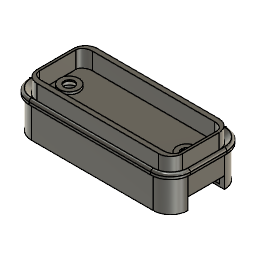
Modul na widgety (Autodesk Fusion 360 design; units mm, degrees)
Autodesk Fusion 360 part; units mm, degrees
note: some values were not read from the file. Set by a fixed rule: which sketch regions a step uses.
sketch "Sketch1" plane through (0, 0, 0) normal (0, 0, 1) x (1, 0, 0)
  line L0 (25, 12.5) -> (-25, 12.5)
  line L1 (-30, 7.5) -> (-30, -7.5)
  line L2 (-25, -12.5) -> (25, -12.5)
  line L3 (30, -7.5) -> (30, 7.5)
  line L4 (-30, 12.5) -> (30, -12.5) construction
  line L5 (-30, -12.5) -> (30, 12.5) construction
  arc A0 (-25, 12.5) -> (-30, 7.5) centre (-25, 7.5) ccw
  arc A1 (30, 7.5) -> (25, 12.5) centre (25, 7.5) ccw
  arc A2 (25, -12.5) -> (30, -7.5) centre (25, -7.5) ccw
  arc A3 (-30, -7.5) -> (-25, -12.5) centre (-25, -7.5) ccw
  circle A4 centre (-24.15, 0) radius 4.85
  line L6 (-30, 0) -> (30, 0) construction
  line L7 (-30, 0) -> (-29, 0) construction
  line L8 (0, 1.75) -> (0, 22.5) construction
  circle A5 centre (24.15, 0) radius 4.85
  circle A6 centre (-24.15, 0) radius 1.75
  circle A7 centre (24.15, 0) radius 1.75
  line L9 (29, -7.5) -> (29, 7.5)
  arc A8 (29, 7.5) -> (25, 11.5) centre (25, 7.5) ccw
  line L10 (25, 11.5) -> (-25, 11.5)
  arc A9 (-25, 11.5) -> (-29, 7.5) centre (-25, 7.5) ccw
  line L11 (-29, 7.5) -> (-29, -7.5)
  arc A10 (-29, -7.5) -> (-25, -11.5) centre (-25, -7.5) ccw
  line L12 (-25, -11.5) -> (25, -11.5)
  arc A11 (25, -11.5) -> (29, -7.5) centre (25, -7.5) ccw
  dimension "d10" = 60
  dimension "d11" = 25
  dimension "d12" = 5
  dimension "d15" = 9.7
  dimension "d16" = 1
  dimension "d17" = 3.5
  dimension "d20" = -1
  constraint horizontal L0
  constraint vertical L1
  constraint horizontal L2
  constraint vertical L3
  constraint midpoint L5 origin
  constraint coincident L4.start L1
  constraint coincident L4.start L0
  constraint tangent L1 A0
  constraint tangent L0 A0
  constraint coincident L5.end L0
  constraint coincident L5.end L3
  constraint tangent L0 A1
  constraint tangent L3 A1
  constraint equal A0 A1
  constraint coincident L4.end L3
  constraint coincident L4.end L2
  constraint tangent L3 A2
  constraint tangent L2 A2
  constraint equal A0 A2
  constraint coincident L5.start L2
  constraint coincident L5.start L1
  constraint tangent L2 A3
  constraint tangent L1 A3
  constraint equal A0 A3
  constraint midpoint L1 L6.start
  constraint midpoint L3 L6.end
  constraint coincident A4.centre L6
  constraint coincident A4 L7.end
  constraint coincident L6 L7.end
  constraint symmetric A4 L8 A5
  constraint concentric A4 A6
  constraint symmetric L8 A6 A7
  measures "d10" distance of L5.end L4.start
  measures "d11" distance of L4.start L5.start
  measures "d12" radius of A0
  measures "d15" diameter of A4
  measures "d16" distance of L6.start L7.end
  measures "d17" diameter of A6
extrude "Extrude1" add sketch "Sketch1" along normal blind 4.6 contours L0 L1 L2 L3 A0 A1 A2 A3 | L9 A8 L10 A9 L11 A10 L12 A11 makes body 1
extrude "Extrude2" add sketch "Sketch1" along normal blind 1 contours A4 | A5 bodies 1
extrude "Extrude3" add sketch "Sketch1" against normal blind 3.9 contours L0 L1 L2 L3 A0 A1 A2 A3 bodies 1
extrude "Extrude4" cut 1 faces at (29, -2.5, -1.3) along direction (1, 0, 0) blind 2 on bodies 1 bodies 1
extrude "Extrude5" cut 1 faces at (-29, 2.5, -1.3) along direction (-1, 0, 0) blind 3 on bodies 1 bodies 1
move_face "OffsetFaces1" offset 4 6 faces at (-27.4726, -10.6442, -2.6) (-8.3333, -11.5, -1.3) (28.2583, -9.8202, -2.6) (27.7603, 10.3949, -2.6) (8.3333, 11.5, -1.3) (-27.7603, 10.3949, -2.6) on bodies 1
copy_body "Body->Comp1" bodies 1 removing the originals makes body 2 in component "spodní část nasazovací"
sketch "Sketch1 (2)" plane through (0, 0, -3.9) normal (0, 0, -1) x (1, 0, 0) in component "spodní část hlavní"
  line L0 (30, -7.5) -> (-30, -7.5)
  arc A0 (-30, -7.5) -> (-25, -12.5) centre (-25, -7.5) ccw
  line L1 (-25, -12.5) -> (25, -12.5)
  arc A1 (25, -12.5) -> (30, -7.5) centre (25, -7.5) ccw
  line L2 (-30, -7.5) -> (30, -7.5)
  line L3 (30, -7.5) -> (30, 7.5)
  line L4 (30, 7.5) -> (-30, 7.5)
  line L5 (-30, 7.5) -> (-30, -7.5)
  circle A2 centre (24.15, 0) radius 1.75
  circle A3 centre (-24.15, 0) radius 1.75
  line L6 (-30, 7.5) -> (30, 7.5)
  arc A4 (30, 7.5) -> (25, 12.5) centre (25, 7.5) ccw
  line L7 (25, 12.5) -> (-25, 12.5)
  arc A5 (-25, 12.5) -> (-30, 7.5) centre (-25, 7.5) ccw
extrude "Extrude1'" add sketch "Sketch1 (2)" along normal blind 1 separate body contours L0 A0 L1 A1 L2 | L0 L2 L3 L4 L5 L6 | L4 L6 A4 L7 A5 | A2 | A3 makes body 3 in component "spodní část hlavní"
sketch "Sketch2" plane through (0, 0, -4.9) normal (0, 0, -1) x (1, 0, 0) in component "spodní část hlavní"
  arc A0 (-25, 12.5) -> (-30, 7.5) centre (-25, 7.5) ccw
  line L0 (-30, 7.5) -> (-30, -7.5)
  arc A1 (-30, -7.5) -> (-25, -12.5) centre (-25, -7.5) ccw
  line L1 (-25, -12.5) -> (25, -12.5)
  arc A2 (25, -12.5) -> (30, -7.5) centre (25, -7.5) ccw
  line L2 (30, -7.5) -> (30, 7.5)
  arc A3 (30, 7.5) -> (25, 12.5) centre (25, 7.5) ccw
  line L3 (25, 12.5) -> (-25, 12.5)
  line L4 (-30.15, 7.5) -> (-30.15, -7.5)
  arc A4 (-30.15, -7.5) -> (-25, -12.65) centre (-25, -7.5) ccw
  line L5 (-25, -12.65) -> (25, -12.65)
  arc A5 (25, -12.65) -> (30.15, -7.5) centre (25, -7.5) ccw
  line L6 (30.15, -7.5) -> (30.15, 7.5)
  arc A6 (30.15, 7.5) -> (25, 12.65) centre (25, 7.5) ccw
  line L7 (25, 12.65) -> (-25, 12.65)
  arc A7 (-25, 12.65) -> (-30.15, 7.5) centre (-25, 7.5) ccw
  line L8 (-32.15, 7.5) -> (-32.15, -7.5)
  arc A8 (-32.15, -7.5) -> (-25, -14.65) centre (-25, -7.5) ccw
  line L9 (-25, -14.65) -> (25, -14.65)
  arc A9 (25, -14.65) -> (32.15, -7.5) centre (25, -7.5) ccw
  line L10 (32.15, -7.5) -> (32.15, 7.5)
  arc A10 (32.15, 7.5) -> (25, 14.65) centre (25, 7.5) ccw
  line L11 (25, 14.65) -> (-25, 14.65)
  arc A11 (-25, 14.65) -> (-32.15, 7.5) centre (-25, 7.5) ccw
  line L12 (30, 7.5) -> (32.15, 7.5)
  line L13 (30, -7.5) -> (32.15, -7.5)
  line L14 (-30, -7.5) -> (-32.15, -7.5)
  line L15 (-30, 7.5) -> (-32.15, 7.5)
  dimension "d30" = 0.15
  dimension "d31" = 2
  constraint coincident L2.end A3.start
  constraint perpendicular L10 L12
  constraint coincident A2.end L2.start
  constraint perpendicular L10 L13
  constraint coincident L0.end A1.start
  constraint perpendicular L8 L14
  constraint coincident A0.end L0.start
  constraint perpendicular L8 L15
extrude "Extrude2'" add sketch "Sketch2" against normal blind 1 contours A0 A3 L3 A6 L7 A7 L12 L15 | L0 L4 L14 L15 | A1 L1 A2 A4 L5 A5 L13 L14 | A6 L7 A7 A10 L11 A11 L12 L15 | L4 L8 L14 L15 | L2 L6 L12 L13 | A4 L5 A5 A8 L9 A9 L13 L14 | L6 L10 L12 L13 bodies 3 in component "spodní část hlavní"
extrude "Extrude3'" add sketch "Sketch2" against normal blind 13.2 contours A6 L7 A7 A10 L11 A11 L12 L15 | L4 L8 L14 L15 | A4 L5 A5 A8 L9 A9 L13 L14 | L6 L10 L12 L13 bodies 3 in component "spodní část hlavní"
sketch "Sketch3" plane through (0, 0, 8.3) normal (0, 0, 1) x (-1, 0, 0) in component "spodní část hlavní"
  arc A0 (30.15, 7.5) -> (25, 12.65) centre (25, 7.5) ccw
  line L0 (30.15, 7.5) -> (30.15, -7.5)
  arc A1 (25, -12.65) -> (30.15, -7.5) centre (25, -7.5) ccw
  line L1 (25, -12.65) -> (-25, -12.65)
  arc A2 (-30.15, -7.5) -> (-25, -12.65) centre (-25, -7.5) ccw
  line L2 (-30.15, -7.5) -> (-30.15, 7.5)
  arc A3 (-25, 12.65) -> (-30.15, 7.5) centre (-25, 7.5) ccw
  line L3 (-25, 12.65) -> (25, 12.65)
  arc A4 (32.15, 7.5) -> (25, 14.65) centre (25, 7.5) ccw
  line L4 (25, 14.65) -> (-25, 14.65)
  arc A5 (-25, 14.65) -> (-32.15, 7.5) centre (-25, 7.5) ccw
  line L5 (-32.15, 7.5) -> (-32.15, -7.5)
  arc A6 (-32.15, -7.5) -> (-25, -14.65) centre (-25, -7.5) ccw
  line L6 (-25, -14.65) -> (25, -14.65)
  arc A7 (25, -14.65) -> (32.15, -7.5) centre (25, -7.5) ccw
  line L7 (32.15, -7.5) -> (32.15, 7.5)
  arc A8 (-33.15, -7.5) -> (-25, -15.65) centre (-25, -7.5) ccw
  line L8 (-25, -15.65) -> (25, -15.65)
  arc A9 (25, -15.65) -> (33.15, -7.5) centre (25, -7.5) ccw
  line L9 (33.15, -7.5) -> (33.15, 7.5)
  arc A10 (33.15, 7.5) -> (25, 15.65) centre (25, 7.5) ccw
  line L10 (25, 15.65) -> (-25, 15.65)
  arc A11 (-25, 15.65) -> (-33.15, 7.5) centre (-25, 7.5) ccw
  line L11 (-33.15, 7.5) -> (-33.15, -7.5)
  dimension "d36" = 1
extrude "Extrude4'" add sketch "Sketch3" along normal blind 2 contours A4 L4 A5 L5 A6 L6 A7 L7 | A8 L8 A9 L9 A10 L10 A11 L11 bodies 3 in component "spodní část hlavní"
chamfer "Chamfer1" distance 2 angle 45 8 edges at (30.15, 0, 10.3) (28.6416, -11.1416, 10.3) (0, -12.65, 10.3) (-28.6416, -11.1416, 10.3) (-30.15, 0, 10.3) (-28.6416, 11.1416, 10.3) (0, 12.65, 10.3) (28.6416, 11.1416, 10.3) on bodies 3 in component "spodní část hlavní"
fillet "Fillet1" radius 1 8 edges at (0, 15.65, 10.3) (-30.7629, 13.2629, 10.3) (-33.15, 0, 10.3) (-30.7629, -13.2629, 10.3) (0, -15.65, 10.3) (30.7629, -13.2629, 10.3) (33.15, 0, 10.3) (30.7629, 13.2629, 10.3) on bodies 3 in component "spodní část hlavní"
extrude "Extrude5'" cut sketch "Sketch1" against normal blind 14 contours A4 | A5 | L9 A8 L10 A9 L11 A10 L12 A11 | A6 | A7 bodies 3 in component "spodní část hlavní"
extrude "Extrude6" add 2 faces at (8.3333, -9.1667, -3.9) (8.3333, 9.1667, -3.9) along direction (0, 0, -1) blind 1 on bodies 2 bodies 3 in component "spodní část hlavní"
sketch "Sketch4" plane through (0, 0, -4.9) normal (0, 0, -1) x (1, 0, 0) in component "spodní část hlavní"
  line L0 (-29, -7.5) -> (-29, 7.5)
  line L1 (-29, 7.5) -> (29, 7.5)
  line L2 (29, 7.5) -> (29, -7.5)
  line L3 (29, -7.5) -> (-29, -7.5)
  arc A0 (-25, 14.65) -> (-32.15, 7.5) centre (-25, 7.5) ccw
  line L4 (-32.15, 7.5) -> (-32.15, -7.5)
  arc A1 (-32.15, -7.5) -> (-25, -14.65) centre (-25, -7.5) ccw
  line L5 (-25, -14.65) -> (25, -14.65)
  arc A2 (25, -14.65) -> (32.15, -7.5) centre (25, -7.5) ccw
  line L6 (32.15, -7.5) -> (32.15, 7.5)
  arc A3 (32.15, 7.5) -> (25, 14.65) centre (25, 7.5) ccw
  line L7 (25, 14.65) -> (-25, 14.65)
  line L8 (-29, -7.5) -> (-32.15, -7.5)
  line L9 (-29, 7.5) -> (-32.15, 7.5)
  line L10 (29, -7.5) -> (32.15, -7.5)
  line L11 (29, 7.5) -> (32.15, 7.5)
  constraint coincident L0.start L3.end
  constraint coincident L4.end A1.start
  constraint coincident L0.end L1.start
  constraint coincident A0.end L4.start
  constraint coincident L2.end L3.start
  constraint coincident A2.end L6.start
  constraint coincident L1.end L2.start
  constraint coincident L6.end A3.start
extrude "Extrude7" cut sketch "Sketch4" against normal blind 4.9 contours L0 L4 L8 L9 | L2 L6 L10 L11 bodies 3 in component "spodní část hlavní"
sketch "Sketch1 (3)" plane through (0, 0, 4.6) normal (0, 0, 1) x (-1, 0, 0) in component "stejná část widgetu"
  circle A0 centre (24.15, 0) radius 4.85
  circle A1 centre (-24.15, 0) radius 4.85
  arc A2 (-30, -7.5) -> (-25, -12.5) centre (-25, -7.5) ccw
  line L0 (-25, -12.5) -> (25, -12.5)
  arc A3 (25, -12.5) -> (30, -7.5) centre (25, -7.5) ccw
  line L1 (30, -7.5) -> (30, 7.5)
  arc A4 (30, 7.5) -> (25, 12.5) centre (25, 7.5) ccw
  line L2 (25, 12.5) -> (-25, 12.5)
  arc A5 (-25, 12.5) -> (-30, 7.5) centre (-25, 7.5) ccw
  line L3 (-30, 7.5) -> (-30, -7.5)
  circle A6 centre (-24.15, 0) radius 3.8
  circle A7 centre (-24.15, 0) radius 2.15
  line L4 (0, -2.5) -> (0, -20)
  circle A8 centre (24.15, 0) radius 2.15
  circle A9 centre (24.15, 0) radius 3.8
  line L5 (-25, -12.45) -> (25, -12.45)
  arc A10 (25, -12.45) -> (29.95, -7.5) centre (25, -7.5) ccw
  line L6 (29.95, -7.5) -> (29.95, 7.5)
  arc A11 (29.95, 7.5) -> (25, 12.45) centre (25, 7.5) ccw
  line L7 (25, 12.45) -> (-25, 12.45)
  arc A12 (-25, 12.45) -> (-29.95, 7.5) centre (-25, 7.5) ccw
  line L8 (-29.95, 7.5) -> (-29.95, -7.5)
  arc A13 (-29.95, -7.5) -> (-25, -12.45) centre (-25, -7.5) ccw
  dimension "d48" = 7.6
  dimension "d49" = 4.3
  dimension "d65" = -0.05
  constraint concentric A1 A6
  constraint concentric A6 A7
  constraint symmetric A6 L4 A9
  constraint symmetric A7 L4 A8
  measures "d48" diameter of A6
  measures "d49" diameter of A7
extrude "Extrude1''" add sketch "Sketch1 (3)" along normal blind 3.2 separate body contours A0 | A1 | A6 | A9 | L5 A10 L6 A11 L7 A12 L8 A13 makes body 4 in component "stejná část widgetu"
chamfer "Chamfer1'" distance 3.2 distance2 1.65 2 edges at (26.1545, -0.7775, 4.6) (-22.1455, -0.7775, 4.6) measured on face at (22.0027, 0.1072, 6.7333) measured on face at (-26.2973, 0.1072, 6.7333) on bodies 4 in component "stejná část widgetu"
sketch "Sketch2 (2)" plane through (0, 0, 4.6) normal (0, 0, -1) x (1, 0, 0) in component "stejná část widgetu"
  circle A0 centre (24.15, 0) radius 3.8
  circle A1 centre (-24.15, 0) radius 3.8
  arc A2 (25, -12.45) -> (29.95, -7.5) centre (25, -7.5) ccw
  line L0 (29.95, -7.5) -> (29.95, 7.5)
  arc A3 (29.95, 7.5) -> (25, 12.45) centre (25, 7.5) ccw
  line L1 (25, 12.45) -> (-25, 12.45)
  arc A4 (-25, 12.45) -> (-29.95, 7.5) centre (-25, 7.5) ccw
  line L2 (-29.95, 7.5) -> (-29.95, -7.5)
  arc A5 (-29.95, -7.5) -> (-25, -12.45) centre (-25, -7.5) ccw
  line L3 (-25, -12.45) -> (25, -12.45)
extrude "Extrude2''" cut sketch "Sketch2 (2)" against normal blind 1 contours A0 | A1 | A2 L0 A3 L1 A4 L2 A5 L3 bodies 4 in component "stejná část widgetu"
extrude "Extrude3''" add 1 faces at (-7.4043, -8.611, 7.8) along direction (0, 0, 1) blind 0.5 on bodies 4 bodies 4 in component "stejná část widgetu"
sketch "Sketch3 (2)" plane through (0, 0, 8.3) normal (0, 0, 1) x (-1, 0, 0) in component "stejná část widgetu"
  circle A0 centre (24.15, 0) radius 2.15
  circle A1 centre (-24.15, 0) radius 2.15
  circle A2 centre (-24.15, 0) radius 4
  line L0 (0, -2.5) -> (0, -20)
  circle A3 centre (24.15, 0) radius 4
  arc A4 (-29.95, -7.5) -> (-25, -12.45) centre (-25, -7.5) ccw
  line L1 (-25, -12.45) -> (25, -12.45)
  arc A5 (25, -12.45) -> (29.95, -7.5) centre (25, -7.5) ccw
  line L2 (29.95, -7.5) -> (29.95, 7.5)
  arc A6 (29.95, 7.5) -> (25, 12.45) centre (25, 7.5) ccw
  line L3 (25, 12.45) -> (-25, 12.45)
  arc A7 (-25, 12.45) -> (-29.95, 7.5) centre (-25, 7.5) ccw
  line L4 (-29.95, 7.5) -> (-29.95, -7.5)
  dimension "d58" = 8
  constraint concentric A1 A2
  constraint symmetric A2 L0 A3
  measures "d58" diameter of A2
extrude "Extrude4''" cut sketch "Sketch3 (2)" against normal blind 1 contours A4 L1 A5 L2 A6 L3 A7 L4 bodies 4 in component "stejná část widgetu"
sketch "Sketch4 (2)" plane through (0, 0, 7.3) normal (0, 0, 1) x (-1, 0, 0) in component "stejná část widgetu"
  circle A0 centre (24.15, 0) radius 4
  circle A1 centre (-24.15, 0) radius 4
  line L0 (-29.95, 7.5) -> (-29.95, -7.5)
  arc A2 (-29.95, -7.5) -> (-25, -12.45) centre (-25, -7.5) ccw
  line L1 (-25, -12.45) -> (25, -12.45)
  arc A3 (25, -12.45) -> (29.95, -7.5) centre (25, -7.5) ccw
  line L2 (29.95, -7.5) -> (29.95, 7.5)
  arc A4 (29.95, 7.5) -> (25, 12.45) centre (25, 7.5) ccw
  line L3 (25, 12.45) -> (-25, 12.45)
  arc A5 (-25, 12.45) -> (-29.95, 7.5) centre (-25, 7.5) ccw
  line L4 (-25, -10.45) -> (25, -10.45)
  line L5 (25, 10.45) -> (-25, 10.45)
  line L6 (-28.95, 7.5) -> (-28.95, -7.5)
  line L7 (28.95, -7.5) -> (28.95, 7.5)
  spline S0 degree 5 poles (-25, 10.45) (-25.2273, 10.45) (-25.6786, 10.4247) (-26.3452, 10.3108) (-27.2024, 10.0207) (-28.141, 9.4513) (-28.6824, 8.8161) (-28.9013, 8.2133) (-28.95, 7.7483) (-28.95, 7.5) knots 0 0 0 0 0 0 0.2 0.4 0.6 0.8 1 1 1 1 1 1
  spline S1 degree 5 poles (-28.95, -7.5) (-28.95, -7.7625) (-28.9031, -8.2507) (-28.6924, -8.8725) (-28.1699, -9.5067) (-27.2532, -10.0523) (-26.3968, -10.3218) (-25.7128, -10.4267) (-25.2404, -10.45) (-25, -10.45) knots 0 0 0 0 0 0 0.2 0.4 0.6 0.8 1 1 1 1 1 1
  spline S2 degree 5 poles (25, -10.45) (25.2273, -10.45) (25.6786, -10.4247) (26.3452, -10.3108) (27.2024, -10.0207) (28.141, -9.4513) (28.6824, -8.8161) (28.9013, -8.2133) (28.95, -7.7483) (28.95, -7.5) knots 0 0 0 0 0 0 0.2 0.4 0.6 0.8 1 1 1 1 1 1
  spline S3 degree 5 poles (28.95, 7.5) (28.95, 7.7625) (28.9031, 8.2507) (28.6924, 8.8725) (28.1699, 9.5067) (27.2532, 10.0523) (26.3968, 10.3218) (25.7128, 10.4267) (25.2404, 10.45) (25, 10.45) knots 0 0 0 0 0 0 0.2 0.4 0.6 0.8 1 1 1 1 1 1
  dimension "d66" = -2
  dimension "d67" = -1
extrude "Extrude5''" add sketch "Sketch4 (2)" along normal blind 7 contours L0 A2 L1 A3 L2 A4 L3 A5 bodies 4 in component "stejná část widgetu"
component "spodní část nasazovací" placed x (1, 0, 0) y (0, 1, 0) z (0, 0, 1) at (0, 0, 0)
component "spodní část hlavní" placed x (1, 0, 0) y (0, 1, 0) z (0, 0, 1) at (0, 0, 0)
component "stejná část widgetu" placed x (1, 0, 0) y (0, 1, 0) z (0, 0, 1) at (0, 0, 0)
equation "d13 = 1 mm + 3.6 mm"
equation "d21 = -8.5 mm + 4.6 mm"
